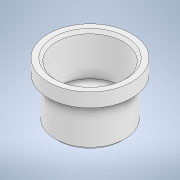
# Autodesk Inventor part: Z_screw_lower_end
Saved by Autodesk Inventor 2020 (Build 240168000, 168)
## iProperties
Created: 2022-03-21
Part Number: Z_screw_lower_end
Material: Tworzywo sztuczne ABS
Document SubType Name: Modeling
Designer: mikoma
Density: 1.06 g/cm^3
Appearance: Gładki — biały
Mass: 17.0242 g
Surface Area: 68.4808 cm^2
Volume: 16.0606 cm^3
Author: mikoma
Autodesk Inventor part; units mm, degrees
ref_plane "YZ Plane" through (0, 0, 0) normal (1, 0, 0) x (0, 1, 0)
ref_plane "XZ Plane" through (0, 0, 0) normal (0, 1, 0) x (-1, 0, 0)
ref_plane "XY Plane" through (0, 0, 0) normal (0, 0, 1) x (1, 0, 0)
sketch "Szkic1" plane through (0, 0, 0) normal (0, 1, 0) x (-1, 0, 0)
  circle A0 centre (0, 0) radius 15
  circle A1 centre (0, 0) radius 12
  circle A2 centre (0, 0) radius 12.5
  circle A3 centre (0, 0) radius 4
  dimension "d0" = 30
  dimension "d1" = 24
  dimension "d2" = 25
  dimension "d12" = 8
  constraints: 4 centre point, 4 coincident
  measures "d0" diameter of A0
  measures "d1" diameter of A1
  measures "d2" diameter of A2
  measures "d12" diameter of A3
extrude "Wyciągnięcie proste1" add sketch "Szkic1" along normal blind 20 contours A0 | A1 | A2 | A3
extrude "Wyciągnięcie proste2" cut sketch "Szkic1" against normal blind 15 from surface at 20 contours A1 | A3
extrude "Wyciągnięcie proste3" cut sketch "Szkic1" along normal blind 15 contours A0
chamfer "Faza1" distance 1 angle 45 2 edges at (12.5, 0, 0) (12, 20, 0)
extrude "Wyciągnięcie proste4" add sketch "Szkic1" along normal blind 8 contours A3
fillet "Zaokrąglenie1" radius 4 1 edges at (4, 8, 0)
